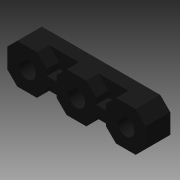
# Autodesk Inventor part: 276-1209
Saved by Autodesk Inventor 2016 (Build 200138000, 138)
## iProperties
Category: Motion
Company: Autodesk Inc.
Created: 2012-04-10
Part Number: 276-1209
Document SubType Name: Modeling
Designer: Autodesk Inc.
Density: 1.425 g/cm^3
Material: Acetal Resin, White
Catalog Web Link: http://www.vexrobotics.com/products/accessories/motion/276-1209.html
Vendor: VEX
Mass: 2.18937 g
Surface Area: 16.163 cm^2
Volume: 1.5364 cm^3
Appearance: Glossy - Black
d65: 0.000 in
d66: 0.000 in
d67: 0.000 in
d68: 0.000 in
d69: 0.000 in
d70: 0.000 in
Author: Autodesk Inc.
Autodesk Inventor part; units mm, degrees
ref_plane "YZ Plane" through (0, 0, 0) normal (1, 0, 0) x (0, 1, 0)
ref_plane "XZ Plane" through (0, 0, 0) normal (0, 1, 0) x (-1, 0, 0)
ref_plane "XY Plane" through (0, 0, 0) normal (0, 0, 1) x (1, 0, 0)
sketch "Sketch1" plane through (0, 0, 0) normal (0, 0, 1) x (1, 0, 0)
  line L0 (-18.9704, 5.6466) -> (16.5896, 5.6466)
  line L1 (16.5896, 5.6466) -> (16.5896, -4.5134)
  line L2 (16.5896, -4.5134) -> (-18.9704, -4.5134)
  line L3 (-18.9704, -4.5134) -> (-18.9704, 5.6466)
  dimension "d0" = 10.16
  dimension "d1" = 35.56
  constraints: 8 end point, 2 parallel, 1 horizontal, 1 perpendicular
  measures "d0" distance of L2.end L0.start
  measures "d1" distance of L1.end L2.end
extrude "Extrusion1" add sketch "Sketch1" along normal blind 3.175
chamfer "Chamfer1" distance 2.54 angle 45 4 edges at (16.5896, 5.6466, 1.5875) (-18.9704, -4.5134, 1.5875) (-18.9704, 5.6466, 1.5875) (16.5896, -4.5134, 1.5875)
sketch "Sketch2" plane through (0, 0, 3.175) normal (0, 0, 1) x (1, 0, 0)
  line L0 (-16.4304, -4.5134) -> (-18.9704, -1.9734) projected
  line L1 (14.0496, -4.5134) -> (-16.4304, -4.5134) projected
  line L2 (16.5896, -1.9734) -> (14.0496, -4.5134) projected
  line L3 (16.5896, 3.1066) -> (16.5896, -1.9734) projected
  line L4 (14.0496, 5.6466) -> (16.5896, 3.1066) projected
  line L5 (-16.4304, 5.6466) -> (14.0496, 5.6466) projected
  line L6 (-18.9704, 3.1066) -> (-16.4304, 5.6466) projected
  line L7 (-18.9704, -1.9734) -> (-18.9704, 3.1066) projected
  line L8 (-18.9704, 3.1066) -> (-16.4304, 5.6466)
  line L9 (-11.3504, 5.6466) -> (-8.8104, 3.1066)
  line L10 (-8.8104, 3.1066) -> (-8.8104, -1.9734)
  line L11 (-8.8104, -1.9734) -> (-11.3504, -4.5134)
  line L12 (-16.4304, -4.5134) -> (-18.9704, -1.9734)
  line L13 (-18.9704, 3.1066) -> (-16.4304, 5.6466)
  line L14 (14.0496, 5.6466) -> (16.5896, 3.1066)
  line L15 (16.5896, -1.9734) -> (14.0496, -4.5134)
  line L16 (8.9696, -4.5134) -> (6.4296, -1.9734)
  line L17 (6.4296, -1.9734) -> (6.4296, 3.1066)
  line L18 (6.4296, 3.1066) -> (8.9696, 5.6466)
  line L19 (-3.7304, 5.6466) -> (1.3496, 5.6466)
  line L20 (1.3496, 5.6466) -> (3.8896, 3.1066)
  line L21 (3.8896, 3.1066) -> (3.8896, -1.9734)
  line L22 (3.8896, -1.9734) -> (1.3496, -4.5134)
  line L23 (-3.7304, -4.5134) -> (-6.2704, -1.9734)
  line L24 (-6.2704, -1.9734) -> (-6.2704, 3.1066)
  line L25 (-6.2704, 3.1066) -> (-3.7304, 5.6466)
  line L26 (-8.8104, 1.5826) -> (-6.2704, 1.5826)
  line L27 (-6.2704, 1.5826) -> (-6.2704, -0.4494)
  line L28 (-6.2704, -0.4494) -> (-8.8104, -0.4494)
  line L29 (-8.8104, -0.4494) -> (-8.8104, 1.5826)
  line L30 (3.8896, 1.5826) -> (6.4296, 1.5826)
  line L31 (6.4296, 1.5826) -> (6.4296, -0.4494)
  line L32 (6.4296, -0.4494) -> (3.8896, -0.4494)
  line L33 (3.8896, -0.4494) -> (3.8896, 1.5826)
  dimension "d7" = 10.16
  dimension "d8" = 2.54
  dimension "d9" = 2.54
  dimension "d10" = 10.16
  dimension "d11" = 2.54
  dimension "d12" = 2.54
  dimension "d13" = 2.54
  dimension "d14" = 2.54
  dimension "d15" = 2.54
  dimension "d16" = 10.16
  dimension "d17" = 2.54
  dimension "d18" = 2.54
  dimension "d19" = 2.032
  dimension "d20" = 4.064
  constraints: 52 end point, 12 perpendicular, 12 point on line, 11 equal length, 2 collinear, 2 horizontal
  measures "d7" distance between parallel lines of L7 L10
  measures "d8" horizontal distance of L9.start L9.end
  measures "d9" horizontal distance of L10.end L11.end
  measures "d10" distance between parallel lines of L21 L24
  measures "d11" distance between parallel lines of L10 L24
  measures "d12" horizontal distance of L21.end L22.end
  measures "d13" horizontal distance of L23.start L23.end
  measures "d14" horizontal distance of L24.end L19.start
  measures "d15" horizontal distance of L19.end L20.end
  measures "d16" distance between parallel lines of L3 L17
  measures "d17" horizontal distance of L17.end L18.end
  measures "d18" horizontal distance of L16.start L16.end
  measures "d19" distance between parallel lines of L28 L26
  measures "d20" distance between parallel lines of L5 L26
extrude "Extrusion2" add sketch "Sketch2" along normal blind 3.175 contours L0 L7 L6 L5 L9 L10 L11 L1 | L23 L24 L25 L5 L20 L21 L22 L1 | L10 L26 L24 L28 | L16 L17 L18 L5 L4 L3 L2 L1 | L21 L30 L17 L32
sketch "Sketch3" plane through (0, 0, 6.35) normal (0, 0, 1) x (1, 0, 0)
  line L0 (3.8896, -0.4494) -> (3.8896, -1.9734) projected
  line L1 (16.5896, 3.1066) -> (16.5896, -1.9734) projected
  line L2 (8.9696, 5.6466) -> (14.0496, 5.6466) projected
  line L3 (-3.7304, 5.6466) -> (1.3496, 5.6466) projected
  line L4 (-16.4304, 5.6466) -> (-11.3504, 5.6466) projected
  line L5 (-18.9704, -1.9734) -> (-18.9704, 3.1066) projected
  line L6 (-15.9859, 2.6621) -> (-11.7949, 2.6621)
  line L7 (-11.7949, 2.6621) -> (-11.7949, -1.5289)
  line L8 (-11.7949, -1.5289) -> (-15.9859, -1.5289)
  line L9 (-15.9859, -1.5289) -> (-15.9859, 2.6621)
  line L10 (-3.2859, 2.6621) -> (0.9051, 2.6621)
  line L11 (0.9051, 2.6621) -> (0.9051, -1.5289)
  line L12 (0.9051, -1.5289) -> (-3.2859, -1.5289)
  line L13 (-3.2859, -1.5289) -> (-3.2859, 2.6621)
  line L14 (9.4141, 2.6621) -> (13.6051, 2.6621)
  line L15 (13.6051, 2.6621) -> (13.6051, -1.5289)
  line L16 (13.6051, -1.5289) -> (9.4141, -1.5289)
  line L17 (9.4141, -1.5289) -> (9.4141, 2.6621)
  point P0 (-13.8904, 0.5666)
  point P1 (-1.1904, 0.5666)
  point P2 (11.5096, 0.5666)
  dimension "d23" = 5.08
  dimension "d24" = 5.08
  dimension "d25" = 5.08
  dimension "d26" = 5.08
  dimension "d27" = 5.08
  dimension "d28" = 5.08
  dimension "d29" = 4.191
  dimension "d30" = 4.191
  dimension "d31" = 4.191
  dimension "d32" = 4.191
  dimension "d33" = 2.0955
  dimension "d34" = 2.0955
  dimension "d35" = 2.0955
  dimension "d36" = 2.0955
  constraints: 24 end point, 6 parallel, 4 collinear, 3 horizontal, 3 perpendicular
  measures "d23" distance from line of L1 point (11.51, 0.567)
  measures "d24" distance from line of L2 point (11.51, 0.567)
  measures "d25" distance from line of L0 point (-1.19, 0.567)
  measures "d26" distance from line of point (-1.19, 0.567) L3
  measures "d27" distance from line of L4 point (-13.89, 0.567)
  measures "d28" distance from line of L5 point (-13.89, 0.567)
  measures "d29" distance of L8.end L6.start
  measures "d30" distance of L6.start L6.end
  measures "d31" distance of L10.start L10.end
  measures "d32" distance of L14.start L14.end
  measures "d33" distance from line of point (11.51, 0.567) L17
  measures "d34" distance from line of L11 point (-1.19, 0.567)
  measures "d35" distance from line of L7 point (-13.89, 0.567)
  measures "d36" distance from line of L8 point (-13.89, 0.567)
extrude "Extrusion3" add sketch "Sketch3" against normal blind 6.985
sketch "Sketch4" plane through (0, 0, 6.35) normal (0, 0, 1) x (1, 0, 0)
  line L0 (8.9696, 5.6466) -> (14.0496, 5.6466) projected
  line L1 (-3.7304, 5.6466) -> (1.3496, 5.6466) projected
  line L2 (-16.4304, 5.6466) -> (-11.3504, 5.6466) projected
  line L3 (-18.9704, -1.9734) -> (-18.9704, 3.1066) projected
  point P0 (-13.8904, 0.5666)
  point P1 (-1.1904, 0.5666)
  point P2 (11.5096, 0.5666)
  dimension "d39" = 5.08
  dimension "d40" = 5.08
  dimension "d41" = 12.7
  dimension "d42" = 12.7
  dimension "d43" = 5.08
  dimension "d44" = 5.08
  measures "d39" distance from line of L3 point (-13.89, 0.567)
  measures "d40" distance from line of point (-13.89, 0.567) L2
  measures "d41" distance of point (-1.19, 0.567) point (-13.89, 0.567)
  measures "d42" distance of point (11.51, 0.567) point (-1.19, 0.567)
  measures "d43" distance from line of L1 point (-1.19, 0.567)
  measures "d44" distance from line of L0 point (11.51, 0.567)
hole "Hole1" at (-13.8904, 0.5666, 6.35) at (-1.1904, 0.5666, 6.35) at (11.5096, 0.5666, 6.35) direction (0, 0, -1) diameter 4.445 depth 19.05 tip angle 118
sketch "Sketch5" plane through (0, 0, 0) normal (0, 0, -1) x (-1, 0, 0)
  line L0 (18.9704, -1.9734) -> (18.9704, 3.1066) projected
  line L1 (16.4304, 5.6466) -> (-14.0496, 5.6466) projected
  line L2 (-16.5896, 3.1066) -> (-16.5896, -1.9734) projected
  line L3 (-14.0496, -4.5134) -> (16.4304, -4.5134) projected
  line L4 (-8.9696, 4.1226) -> (-2.6196, 4.1226)
  line L5 (-2.6196, 4.1226) -> (-2.6196, -2.9894)
  line L6 (-2.6196, -2.9894) -> (-8.9696, -2.9894)
  line L7 (-8.9696, -2.9894) -> (-8.9696, 4.1226)
  line L8 (5.0004, 4.1226) -> (11.3504, 4.1226)
  line L9 (11.3504, 4.1226) -> (11.3504, -2.9894)
  line L10 (11.3504, -2.9894) -> (5.0004, -2.9894)
  line L11 (5.0004, -2.9894) -> (5.0004, 4.1226)
  dimension "d52" = 7.62
  dimension "d53" = 7.62
  dimension "d54" = 7.62
  dimension "d55" = 6.35
  dimension "d56" = 1.524
  dimension "d57" = 1.524
  constraints: 16 end point, 4 parallel, 2 collinear, 2 horizontal, 2 perpendicular
  measures "d52" distance between parallel lines of L7 L2
  measures "d53" distance between parallel lines of L0 L9
  measures "d54" distance between parallel lines of L11 L5
  measures "d55" distance of L4.start L4.end
  measures "d56" distance between parallel lines of L1 L4
  measures "d57" distance between parallel lines of L3 L6
extrude "Extrusion4" cut sketch "Sketch5" against normal blind 1.905
sketch "Sketch6" plane through (0, 0, 6.35) normal (0, 0, 1) x (1, 0, 0)
  circle A0 centre (-13.8904, 0.5666) radius 2.2225 projected
  circle A1 centre (-13.8904, 0.5666) radius 2.2225
  point P0 (0, 0)
  constraints: 1 centre point, 1 coincident, 1 concentric
surface extrude "ExtrusionSrf1" sketch "Sketch6" against normal up to surface (6.35 mm away) shown no curves A0
pattern_linear "Rectangular Pattern1" count 3 spacing 12.7 along (1, 0, 0) of "ExtrusionSrf1"
body "Solid1"
body "Srf1"
body "Srf2"
body "Srf3"
